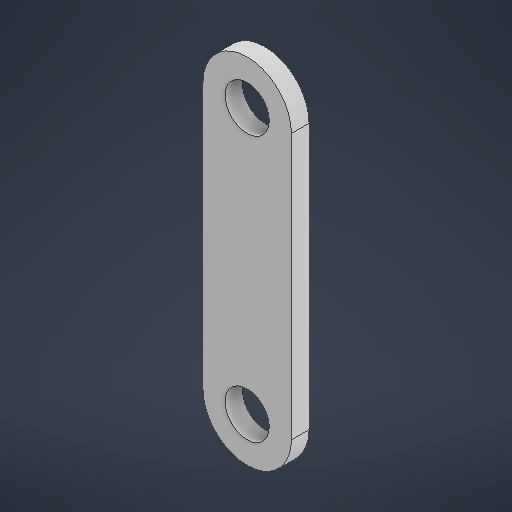
# Autodesk Inventor part: arm
Saved by Autodesk Inventor 2026.1 (Build 301233000, 233)
## iProperties
Created: 2026-06-10
Part Number: arm
Material: Generic
Document SubType Name: Modeling
Designer: share
Density: 1 g/cm^3
Appearance: Default
Author: share
Autodesk Inventor part; units mm, degrees
ref_plane "YZ Plane" through (0, 0, 0) normal (1, 0, 0) x (0, 1, 0)
ref_plane "XZ Plane" through (0, 0, 0) normal (0, 1, 0) x (-1, 0, 0)
ref_plane "XY Plane" through (0, 0, 0) normal (0, 0, 1) x (1, 0, 0)
sketch "Sketch1" plane through (0, 0, 0) normal (0, 0, 1) x (1, 0, 0)
  circle A0 centre (0, 0) radius 6.35
  circle A1 centre (0, 0) radius 3.175
  line L0 (0, 0) -> (0, 38.1)
  circle A2 centre (0, 38.1) radius 6.35
  circle A3 centre (0, 38.1) radius 3.175
  line L1 (-6.35, 38.1) -> (-6.35, 0)
  line L2 (6.35, 0) -> (6.35, 38.1)
  dimension "d1" = 12.7
  dimension "d2" = 6.35
  dimension "d4" = 38.1
  constraints: 6 end point, 4 centre point, 4 coincident, 4 point on circle, 2 equal radius, 2 parallel, 2 tangent, 1 vertical
  measures "d1" diameter of A2
  measures "d2" diameter of A3
  measures "d4" distance of L0.start L0.end
extrude "Extrusion1" add sketch "Sketch1" along normal blind 2.54
body "Solid1"
